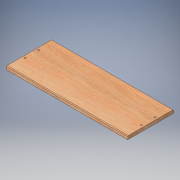
# Autodesk Inventor part: cabinet-bottom
Saved by Autodesk Inventor 2016 (Build 200138000, 138)
## iProperties
Created: 2015-10-24
Part Number: cabinet-bottom
Material: Wood (Birch)
Document SubType Name: Modeling
Designer: jeremyhale
Density: 0.55 g/cm^3
Appearance: Birch - Natural Polished
Mass: 1280.63 g
Surface Area: 2729.67 cm^2
Volume: 2328.42 cm^3
Author: jeremyhale
Autodesk Inventor part; units mm, degrees
ref_plane "YZ Plane" through (0, 0, 0) normal (1, 0, 0) x (0, 1, 0)
ref_plane "XZ Plane" through (0, 0, 0) normal (0, 1, 0) x (-1, 0, 0)
ref_plane "XY Plane" through (0, 0, 0) normal (0, 0, 1) x (1, 0, 0)
sketch "Sketch1" plane through (0, 0, 0) normal (0, 1, 0) x (-1, 0, 0)
  line L0 (285.8, 107.95) -> (-285.8, 107.95)
  line L1 (-285.8, 107.95) -> (-285.8, -107.95)
  line L2 (-285.8, -107.95) -> (285.8, -107.95)
  line L3 (285.8, -107.95) -> (285.8, 107.95)
  line L4 (285.8, 107.95) -> (-285.8, -107.95) construction
  line L5 (-285.8, 107.95) -> (285.8, -107.95) construction
  point P0 (0, 0)
  dimension "length" = 571.6
  dimension "width" = 215.9
  constraints: 12 end point, 2 midpoint, 2 parallel, 1 horizontal, 1 perpendicular
  measures "length" distance of L2.end L1.end
  measures "width" distance of L1.end L0.end
extrude "Extrusion1" add sketch "Sketch1" along normal blind 19
chamfer "Chamfer1" distance 3.175 angle 45 4 edges at (0, 0, 107.95) (0, 0, -107.95) (285.8, 0, 0) (-285.8, 0, 0)
chamfer "Chamfer2" distance 3.175 angle 45 2 edges at (0, 19, 107.95) (0, 19, -107.95)
sketch "Sketch10" plane through (0, 0, 0) normal (0, -1, 0) x (1, 0, 0)
  point P0 (273.8937, 31.4375)
hole "Hole9" at (273.8937, 0, 31.4375) direction (0, 1, 0) diameter 6.6 depth 19
sketch "Sketch11" plane through (0, 0, 0) normal (0, -1, 0) x (1, 0, 0)
  point P0 (273.8937, -32.0625)
hole "Hole11" at (273.8937, 0, -32.0625) direction (0, 1, 0) diameter 7 depth 19
sketch "Sketch12" plane through (0, 0, 0) normal (0, -1, 0) x (1, 0, 0)
  point P0 (-273.8938, 31.4375)
hole "Hole13" at (-273.8938, 0, 31.4375) direction (0, 1, 0) diameter 6.6 depth 19
sketch "Sketch13" plane through (0, 0, 0) normal (0, -1, 0) x (1, 0, 0)
  point P0 (-273.8938, -32.0625)
hole "Hole15" at (-273.8938, 0, -32.0625) direction (0, 1, 0) diameter 6.6 depth 19
body "Solid1"
